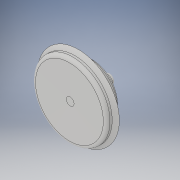
# Autodesk Inventor part: Junk Part Bolt
Saved by Autodesk Inventor 2017 (Build 210142000, 142)
## iProperties
Created: 2017-05-17
Part Number: Junk Part Bolt
Material: Generic
Document SubType Name: Modeling
Designer: User
Density: 1 g/cm^3
Appearance: Default
Author: User
Autodesk Inventor part; units mm, degrees
ref_plane "YZ Plane" through (0, 0, 0) normal (1, 0, 0) x (0, 1, 0)
ref_plane "XZ Plane" through (0, 0, 0) normal (0, 1, 0) x (-1, 0, 0)
ref_plane "XY Plane" through (0, 0, 0) normal (0, 0, 1) x (1, 0, 0)
sketch "Sketch1" plane through (0, 0, 0) normal (0, 1, 0) x (-1, 0, 0)
  line L0 (1.4852, 5.9232) -> (14.181, 6.2487)
  line L1 (14.181, 6.2487) -> (14.2348, 4.1513)
  line L2 (14.2348, 4.1513) -> (15.6087, 2.8286)
  line L3 (15.6087, 2.8286) -> (8.2315, 2.8286)
  line L4 (8.2315, 2.8286) -> (11.577, -0.3921)
  line L5 (11.577, -0.3921) -> (9.5233, -2.5254)
  line L6 (9.5233, -2.5254) -> (8.1474, 0)
  line L7 (8.1474, 0) -> (8.275, -4.9753)
  line L8 (8.275, -4.9753) -> (1.8442, 1.2156)
  line L9 (1.8442, 1.2156) -> (2.1238, -9.6904)
  line L10 (2.1238, -9.6904) -> (0, -9.3364)
  line L11 (0, -9.3364) -> (0, 5.9232)
  line L12 (1.4852, 5.9232) -> (0, 5.9232)
  point P0 (0, 0)
  dimension "d0" = 12.7
  constraints: 26 end point, 3 parallel, 3 perpendicular, 2 horizontal, 1 vertical
  measures "d0" distance of L0.start L0.end
revolve "Revolution1" add sketch "Sketch1" angle 360 about axis through (0, 0, -9.3364) along (0, 0, 1)
fillet "Fillet1" radius 1.27 4 edges at (11.577, 0, -0.3921) (14.181, 0, 6.2487) (2.1238, 0, -9.6904) (8.275, 0, -4.9753)
body "Solid1"
